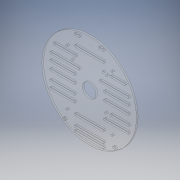
# Autodesk Inventor part: TopPlate
Saved by Autodesk Inventor 2018 (Build 220112000, 112)
## iProperties
Created: 2018-01-11
Part Number: TopPlate
Material: Polycarbonate, Clear
Document SubType Name: Modeling
Designer: Kyle
Density: 1.2 g/cm^3
Appearance: Polycarbonate - Clear
Author: Kyle
Autodesk Inventor part; units mm, degrees
ref_plane "YZ Plane" through (0, 0, 0) normal (1, 0, 0) x (0, 1, 0)
ref_plane "XZ Plane" through (0, 0, 0) normal (0, 1, 0) x (-1, 0, 0)
ref_plane "XY Plane" through (0, 0, 0) normal (0, 0, 1) x (1, 0, 0)
sketch "Sketch1" plane through (0, 0, 0) normal (0, 0, 1) x (1, 0, 0)
  circle A0 centre (0, 0) radius 69.85
  dimension "d0" = 139.7
  constraints: 1 centre point, 1 coincident
  measures "d0" diameter of A0
extrude "Extrusion1" add sketch "Sketch1" along normal blind 2.54
sketch "Sketch2" plane through (0, 0, 2.54) normal (0, 0, 1) x (1, 0, 0)
  circle A0 centre (0, 0) radius 10.16
  dimension "d3" = 20.32
  constraints: 1 centre point, 1 coincident
  measures "d3" diameter of A0
extrude "Extrusion2" cut sketch "Sketch2" against normal blind 2.54
sketch "Sketch3" plane through (0, 0, 2.54) normal (0, 0, 1) x (1, 0, 0)
  circle A0 centre (0, 0) radius 69.85 projected
  line L0 (-20.6375, 48.26) -> (20.6375, 48.26)
  line L1 (22.225, 46.6725) -> (22.225, 46.6725)
  line L2 (20.6375, 45.085) -> (-20.6375, 45.085)
  line L3 (-22.225, 46.6725) -> (-22.225, 46.6725)
  line L4 (14.9225, 63.5) -> (20.6375, 63.5)
  line L5 (22.225, 61.9125) -> (22.225, 61.9125)
  line L6 (20.6375, 60.325) -> (14.9225, 60.325)
  line L7 (13.335, 61.9125) -> (13.335, 61.9125)
  line L8 (-14.9225, 60.325) -> (-20.6375, 60.325)
  line L9 (-22.225, 61.9125) -> (-22.225, 61.9125)
  line L10 (-20.6375, 63.5) -> (-14.9225, 63.5)
  line L11 (-13.335, 61.9125) -> (-13.335, 61.9125)
  arc A1 (20.6375, 45.085) -> (22.225, 46.6725) centre (20.6375, 46.6725) ccw
  arc A2 (22.225, 46.6725) -> (20.6375, 48.26) centre (20.6375, 46.6725) ccw
  circle A3 centre (20.6375, 33.9725) radius 1.5875
  line L12 (32.7025, 35.56) -> (52.3875, 35.56)
  line L13 (53.975, 33.9725) -> (53.975, 33.9725)
  line L14 (52.3875, 32.385) -> (32.7025, 32.385)
  line L15 (31.115, 33.9725) -> (31.115, 33.9725)
  circle A4 centre (33.655, 40.9575) radius 1.5875
  circle A5 centre (25.7175, 32.0675) radius 1.5875
  circle A6 centre (-33.02, 40.9575) radius 1.5875
  line L16 (-51.7525, 35.56) -> (-20.6375, 35.56)
  line L17 (-19.05, 33.9725) -> (-19.05, 33.9725)
  line L18 (-20.6375, 32.385) -> (-51.7525, 32.385)
  line L19 (-53.34, 33.9725) -> (-53.34, 33.9725)
  arc A7 (-20.6375, 48.26) -> (-22.225, 46.6725) centre (-20.6375, 46.6725) ccw
  arc A8 (-22.225, 46.6725) -> (-20.6375, 45.085) centre (-20.6375, 46.6725) ccw
  arc A9 (-20.6375, 32.385) -> (-19.05, 33.9725) centre (-20.6375, 33.9725) ccw
  arc A10 (-19.05, 33.9725) -> (-20.6375, 35.56) centre (-20.6375, 33.9725) ccw
  circle A11 centre (-25.4, 26.3525) radius 1.5875
  arc A12 (-22.225, 61.9125) -> (-20.6375, 60.325) centre (-20.6375, 61.9125) ccw
  arc A13 (-20.6375, 63.5) -> (-22.225, 61.9125) centre (-20.6375, 61.9125) ccw
  arc A14 (-13.335, 61.9125) -> (-14.9225, 63.5) centre (-14.9225, 61.9125) ccw
  arc A15 (-14.9225, 60.325) -> (-13.335, 61.9125) centre (-14.9225, 61.9125) ccw
  arc A16 (14.9225, 63.5) -> (13.335, 61.9125) centre (14.9225, 61.9125) ccw
  arc A17 (13.335, 61.9125) -> (14.9225, 60.325) centre (14.9225, 61.9125) ccw
  arc A18 (20.6375, 60.325) -> (22.225, 61.9125) centre (20.6375, 61.9125) ccw
  arc A19 (22.225, 61.9125) -> (20.6375, 63.5) centre (20.6375, 61.9125) ccw
  arc A20 (-51.7525, 35.56) -> (-53.34, 33.9725) centre (-51.7525, 33.9725) ccw
  arc A21 (-53.34, 33.9725) -> (-51.7525, 32.385) centre (-51.7525, 33.9725) ccw
  arc A22 (32.7025, 35.56) -> (31.115, 33.9725) centre (32.7025, 33.9725) ccw
  arc A23 (31.115, 33.9725) -> (32.7025, 32.385) centre (32.7025, 33.9725) ccw
  arc A24 (52.3875, 32.385) -> (53.975, 33.9725) centre (52.3875, 33.9725) ccw
  arc A25 (53.975, 33.9725) -> (52.3875, 35.56) centre (52.3875, 33.9725) ccw
  line L20 (-56.8325, 21.59) -> (-15.5575, 21.59)
  line L21 (-13.97, 20.0025) -> (-13.97, 20.0025)
  line L22 (-15.5575, 18.415) -> (-56.8325, 18.415)
  line L23 (-58.42, 20.0025) -> (-58.42, 20.0025)
  line L24 (-57.15, 11.43) -> (-22.225, 11.43)
  line L25 (-20.6375, 9.8425) -> (-20.6375, 9.8425)
  line L26 (-22.225, 8.255) -> (-57.15, 8.255)
  line L27 (-58.7375, 9.8425) -> (-58.7375, 9.8425)
  line L28 (-57.15, 0) -> (-22.225, 0)
  line L29 (-20.6375, -1.5875) -> (-20.6375, -1.5875)
  line L30 (-22.225, -3.175) -> (-57.15, -3.175)
  line L31 (-58.7375, -1.5875) -> (-58.7375, -1.5875)
  line L32 (-57.15, -13.97) -> (-22.225, -13.97)
  line L33 (-20.6375, -15.5575) -> (-20.6375, -15.5575)
  line L34 (-22.225, -17.145) -> (-57.15, -17.145)
  line L35 (-58.7375, -15.5575) -> (-58.7375, -15.5575)
  line L36 (-57.15, -24.13) -> (-22.225, -24.13)
  line L37 (-20.6375, -25.7175) -> (-20.6375, -25.7175)
  line L38 (-22.225, -27.305) -> (-57.15, -27.305)
  line L39 (-58.7375, -25.7175) -> (-58.7375, -25.7175)
  arc A26 (-56.8325, 21.59) -> (-58.42, 20.0025) centre (-56.8325, 20.0025) ccw
  arc A27 (-58.42, 20.0025) -> (-56.8325, 18.415) centre (-56.8325, 20.0025) ccw
  arc A28 (-15.5575, 18.415) -> (-13.97, 20.0025) centre (-15.5575, 20.0025) ccw
  arc A29 (-13.97, 20.0025) -> (-15.5575, 21.59) centre (-15.5575, 20.0025) ccw
  arc A30 (-57.15, 11.43) -> (-58.7375, 9.8425) centre (-57.15, 9.8425) ccw
  arc A31 (-58.7375, 9.8425) -> (-57.15, 8.255) centre (-57.15, 9.8425) ccw
  arc A32 (-22.225, 8.255) -> (-20.6375, 9.8425) centre (-22.225, 9.8425) ccw
  arc A33 (-20.6375, 9.8425) -> (-22.225, 11.43) centre (-22.225, 9.8425) ccw
  arc A34 (-58.7375, -1.5875) -> (-57.15, -3.175) centre (-57.15, -1.5875) ccw
  arc A35 (-57.15, 0) -> (-58.7375, -1.5875) centre (-57.15, -1.5875) ccw
  arc A36 (-20.6375, -1.5875) -> (-22.225, 0) centre (-22.225, -1.5875) ccw
  arc A37 (-22.225, -3.175) -> (-20.6375, -1.5875) centre (-22.225, -1.5875) ccw
  arc A38 (-20.6375, -15.5575) -> (-22.225, -13.97) centre (-22.225, -15.5575) ccw
  arc A39 (-22.225, -17.145) -> (-20.6375, -15.5575) centre (-22.225, -15.5575) ccw
  arc A40 (-58.7375, -15.5575) -> (-57.15, -17.145) centre (-57.15, -15.5575) ccw
  arc A41 (-57.15, -13.97) -> (-58.7375, -15.5575) centre (-57.15, -15.5575) ccw
  arc A42 (-57.15, -24.13) -> (-58.7375, -25.7175) centre (-57.15, -25.7175) ccw
  arc A43 (-58.7375, -25.7175) -> (-57.15, -27.305) centre (-57.15, -25.7175) ccw
  arc A44 (-22.225, -27.305) -> (-20.6375, -25.7175) centre (-22.225, -25.7175) ccw
  arc A45 (-20.6375, -25.7175) -> (-22.225, -24.13) centre (-22.225, -25.7175) ccw
  arc A46 (22.733, -24.13) -> (21.1455, -25.7175) centre (22.733, -25.7175) ccw
  arc A47 (21.1455, -25.7175) -> (22.733, -27.305) centre (22.733, -25.7175) ccw
  line L40 (58.928, 20.0025) -> (58.928, 20.0025)
  arc A48 (21.1455, 9.8425) -> (22.733, 8.255) centre (22.733, 9.8425) ccw
  line L41 (22.733, -3.175) -> (57.658, -3.175)
  line L42 (57.658, 0) -> (22.733, 0)
  arc A49 (57.658, -3.175) -> (59.2455, -1.5875) centre (57.658, -1.5875) ccw
  arc A50 (59.2455, -1.5875) -> (57.658, 0) centre (57.658, -1.5875) ccw
  line L43 (22.733, 8.255) -> (57.658, 8.255)
  arc A51 (57.658, 8.255) -> (59.2455, 9.8425) centre (57.658, 9.8425) ccw
  line L44 (57.658, 11.43) -> (22.733, 11.43)
  arc A52 (59.2455, 9.8425) -> (57.658, 11.43) centre (57.658, 9.8425) ccw
  arc A53 (57.3405, 18.415) -> (58.928, 20.0025) centre (57.3405, 20.0025) ccw
  line L45 (16.0655, 18.415) -> (57.3405, 18.415)
  line L46 (57.3405, 21.59) -> (16.0655, 21.59)
  arc A54 (22.733, 11.43) -> (21.1455, 9.8425) centre (22.733, 9.8425) ccw
  arc A55 (21.1455, -1.5875) -> (22.733, -3.175) centre (22.733, -1.5875) ccw
  arc A56 (14.478, 20.0025) -> (16.0655, 18.415) centre (16.0655, 20.0025) ccw
  line L47 (21.1455, 9.8425) -> (21.1455, 9.8425)
  line L48 (14.478, 20.0025) -> (14.478, 20.0025)
  arc A57 (16.0655, 21.59) -> (14.478, 20.0025) centre (16.0655, 20.0025) ccw
  line L49 (21.1455, -25.7175) -> (21.1455, -25.7175)
  line L50 (59.2455, -25.7175) -> (59.2455, -25.7175)
  arc A58 (57.658, -27.305) -> (59.2455, -25.7175) centre (57.658, -25.7175) ccw
  line L51 (57.658, -24.13) -> (22.733, -24.13)
  line L52 (22.733, -27.305) -> (57.658, -27.305)
  line L53 (21.1455, -1.5875) -> (21.1455, -1.5875)
  arc A59 (22.733, 0) -> (21.1455, -1.5875) centre (22.733, -1.5875) ccw
  line L54 (59.2455, -15.5575) -> (59.2455, -15.5575)
  arc A60 (59.2455, -25.7175) -> (57.658, -24.13) centre (57.658, -25.7175) ccw
  line L55 (59.2455, -1.5875) -> (59.2455, -1.5875)
  line L56 (59.2455, 9.8425) -> (59.2455, 9.8425)
  arc A61 (58.928, 20.0025) -> (57.3405, 21.59) centre (57.3405, 20.0025) ccw
  line L57 (32.258, -17.145) -> (57.658, -17.145)
  line L58 (59.2455, -15.5575) -> (59.2455, -15.5575)
  line L59 (57.658, -13.97) -> (32.258, -13.97)
  line L60 (30.6705, -15.5575) -> (30.6705, -15.5575)
  arc A62 (30.6705, -15.5575) -> (32.258, -17.145) centre (32.258, -15.5575) ccw
  arc A63 (32.258, -13.97) -> (30.6705, -15.5575) centre (32.258, -15.5575) ccw
  arc A64 (57.658, -17.145) -> (59.2455, -15.5575) centre (57.658, -15.5575) ccw
  arc A65 (59.2455, -15.5575) -> (57.658, -13.97) centre (57.658, -15.5575) ccw
  circle A66 centre (24.3205, -16.8275) radius 1.5875
  circle A67 centre (33.655, -40.9575) radius 1.5875
  circle A68 centre (-33.02, -40.9575) radius 1.5875
  line L61 (-20.6375, -39.37) -> (20.6375, -39.37)
  line L62 (22.225, -40.9575) -> (22.225, -40.9575)
  line L63 (20.6375, -42.545) -> (-20.6375, -42.545)
  line L64 (-22.225, -40.9575) -> (-22.225, -40.9575)
  line L65 (-20.6375, -54.61) -> (20.6375, -54.61)
  line L66 (22.225, -56.1975) -> (22.225, -56.1975)
  line L67 (20.6375, -57.785) -> (-20.6375, -57.785)
  line L68 (-22.225, -56.1975) -> (-22.225, -56.1975)
  line L69 (-20.6375, -60.96) -> (20.6375, -60.96)
  line L70 (22.225, -62.5475) -> (22.225, -62.5475)
  line L71 (20.6375, -64.135) -> (-20.6375, -64.135)
  line L72 (-22.225, -62.5475) -> (-22.225, -62.5475)
  line L73 (35.8775, -53.34) -> (37.7825, -53.34)
  line L74 (39.37, -54.9275) -> (39.37, -54.9275)
  line L75 (37.7825, -56.515) -> (35.8775, -56.515)
  line L76 (34.29, -54.9275) -> (34.29, -54.9275)
  line L77 (-37.7825, -53.34) -> (-35.8775, -53.34)
  line L78 (-34.29, -54.9275) -> (-34.29, -54.9275)
  line L79 (-35.8775, -56.515) -> (-37.7825, -56.515)
  line L80 (-39.37, -54.9275) -> (-39.37, -54.9275)
  arc A69 (-20.6375, -39.37) -> (-22.225, -40.9575) centre (-20.6375, -40.9575) ccw
  arc A70 (-22.225, -40.9575) -> (-20.6375, -42.545) centre (-20.6375, -40.9575) ccw
  arc A71 (20.6375, -42.545) -> (22.225, -40.9575) centre (20.6375, -40.9575) ccw
  arc A72 (22.225, -40.9575) -> (20.6375, -39.37) centre (20.6375, -40.9575) ccw
  arc A73 (22.225, -56.1975) -> (20.6375, -54.61) centre (20.6375, -56.1975) ccw
  arc A74 (20.6375, -57.785) -> (22.225, -56.1975) centre (20.6375, -56.1975) ccw
  arc A75 (-22.225, -56.1975) -> (-20.6375, -57.785) centre (-20.6375, -56.1975) ccw
  arc A76 (-20.6375, -54.61) -> (-22.225, -56.1975) centre (-20.6375, -56.1975) ccw
  arc A77 (-22.225, -62.5475) -> (-20.6375, -64.135) centre (-20.6375, -62.5475) ccw
  arc A78 (-20.6375, -60.96) -> (-22.225, -62.5475) centre (-20.6375, -62.5475) ccw
  arc A79 (22.225, -62.5475) -> (20.6375, -60.96) centre (20.6375, -62.5475) ccw
  arc A80 (20.6375, -64.135) -> (22.225, -62.5475) centre (20.6375, -62.5475) ccw
  arc A81 (34.29, -54.9275) -> (35.8775, -56.515) centre (35.8775, -54.9275) ccw
  arc A82 (35.8775, -53.34) -> (34.29, -54.9275) centre (35.8775, -54.9275) ccw
  arc A83 (39.37, -54.9275) -> (37.7825, -53.34) centre (37.7825, -54.9275) ccw
  arc A84 (37.7825, -56.515) -> (39.37, -54.9275) centre (37.7825, -54.9275) ccw
  arc A85 (-35.8775, -56.515) -> (-34.29, -54.9275) centre (-35.8775, -54.9275) ccw
  arc A86 (-34.29, -54.9275) -> (-35.8775, -53.34) centre (-35.8775, -54.9275) ccw
  arc A87 (-37.7825, -53.34) -> (-39.37, -54.9275) centre (-37.7825, -54.9275) ccw
  arc A88 (-39.37, -54.9275) -> (-37.7825, -56.515) centre (-37.7825, -54.9275) ccw
  point P0 (0, 69.85)
  point P1 (69.85, 0)
  point P2 (0, -69.85)
  point P3 (-69.85, 0)
  point P4 (22.225, 45.085)
  point P5 (22.225, 48.26)
  point P6 (-22.225, 45.085)
  point P7 (22.225, 60.325)
  point P8 (22.225, 63.5)
  point P9 (13.335, 60.325)
  point P10 (-13.335, 60.325)
  point P11 (-22.225, 63.5)
  point P12 (-22.225, 60.325)
  point P13 (53.975, 32.385)
  point P14 (53.975, 35.56)
  point P15 (31.115, 32.385)
  point P16 (-19.05, 32.385)
  point P17 (-19.05, 35.56)
  point P18 (-53.34, 32.385)
  point P19 (-13.97, 18.415)
  point P20 (-13.97, 21.59)
  point P21 (-58.42, 18.415)
  point P22 (-20.6375, 8.255)
  point P23 (-20.6375, 11.43)
  point P24 (-58.7375, 8.255)
  point P25 (-20.6375, -3.175)
  point P26 (-20.6375, 0)
  point P27 (-58.7375, -3.175)
  point P28 (-20.6375, -17.145)
  point P29 (-20.6375, -13.97)
  point P30 (-58.7375, -17.145)
  point P31 (-20.6375, -27.305)
  point P32 (-20.6375, -24.13)
  point P33 (-58.7375, -27.305)
  point P34 (14.478, 20.0025)
  point P35 (59.2455, -3.175)
  point P36 (59.2455, 8.255)
  point P37 (58.928, 18.415)
  point P38 (21.1455, -24.13)
  point P39 (30.6705, -17.145)
  point P40 (21.1455, 0)
  point P41 (21.1455, 8.255)
  point P42 (14.478, 18.415)
  point P43 (14.478, 21.59)
  point P44 (21.1455, -27.305)
  point P45 (59.2455, -27.305)
  point P46 (21.1455, -3.175)
  point P47 (59.2455, -17.145)
  point P48 (21.1455, 11.43)
  point P49 (30.6705, -17.145)
  point P50 (-22.225, -39.37)
  point P51 (22.225, -39.37)
  point P52 (-22.225, -54.61)
  point P53 (22.225, -54.61)
  point P54 (-22.225, -60.96)
  point P55 (22.225, -60.96)
  point P56 (34.29, -53.34)
  point P57 (39.37, -56.515)
  point P58 (39.37, -53.34)
  point P59 (-39.37, -53.34)
  point P60 (-34.29, -53.34)
  dimension "d6" = 44.45
  dimension "d7" = 3.175
  dimension "d8" = 22.225
  dimension "d9" = 21.59
  dimension "d10" = 8.89
  dimension "d11" = 8.89
  dimension "d12" = 3.175
  dimension "d13" = 3.175
  dimension "d14" = 12.065
  dimension "d15" = 12.065
  dimension "d16" = 1.5875
  dimension "d17" = 3.175
  dimension "d18" = 11.1125
  dimension "d19" = 3.175
  dimension "d20" = 22.86
  dimension "d21" = 10.4775
  dimension "d22" = 3.175
  dimension "d23" = 5.3975
  dimension "d24" = 2.54
  dimension "d25" = 3.175
  dimension "d26" = 5.08
  dimension "d27" = 1.905
  dimension "d28" = 3.175
  dimension "d29" = 3.175
  dimension "d30" = 34.29
  dimension "d31" = 1.5875
  dimension "d32" = 1.5875
  dimension "d33" = 1.5875
  dimension "d34" = 0
  dimension "d35" = 13.97
  dimension "d36" = 3.175
  dimension "d37" = 6.0325
  dimension "d38" = 6.35
  dimension "d39" = 1.5875
  dimension "d40" = 3.175
  dimension "d41" = 44.45
  dimension "d42" = 5.08
  dimension "d43" = 10.795
  dimension "d44" = 3.175
  dimension "d45" = 38.1
  dimension "d46" = 6.985
  dimension "d47" = 3.175
  dimension "d48" = 38.1
  dimension "d49" = 3.175
  dimension "d50" = 38.1
  dimension "d51" = 3.175
  dimension "d52" = 38.1
  dimension "d53" = 8.255
  dimension "d54" = 10.795
  dimension "d55" = 6.985
  dimension "d56" = 1.5875
  dimension "d57" = 28.448
  dimension "d74" = 28.575
  dimension "d75" = 1.5875
  dimension "d76" = 3.175
  dimension "d77" = 6.35
  dimension "d78" = 1.27
  dimension "d79" = 44.45
  dimension "d80" = 22.225
  dimension "d81" = 44.45
  dimension "d82" = 44.45
  dimension "d83" = 39.37
  dimension "d84" = 12.065
  dimension "d85" = 3.175
  constraints: 164 point on circle, 162 end point, 128 tangent, 109 point on line, 88 centre point, 56 equal radius, 32 parallel, 16 horizontal, 16 perpendicular, 2 collinear, 2 symmetric about line, 1 coincident, 1 vertical, 7 other
  measures "d6" distance of point (22.225, 45.085) point (-22.225, 45.085)
  measures "d7" distance of point (22.225, 48.26) point (22.225, 45.085)
  measures "d8" distance from line of A0.start L1
  measures "d9" distance from line of A0.start L0
  measures "d10" distance of point (22.225, 60.325) point (13.335, 60.325)
  measures "d11" distance of point (-13.335, 60.325) point (-22.225, 60.325)
  measures "d12" distance of point (-22.225, 60.325) point (-22.225, 63.5)
  measures "d13" distance of point (22.225, 63.5) point (22.225, 60.325)
  measures "d14" distance between parallel lines of L0 L6
  measures "d15" distance between parallel lines of L8 L0
  measures "d16" radius of A1
  measures "d17" diameter of A3
  measures "d18" distance from line of A3.centre L2
  measures "d19" distance of point (53.975, 35.56) point (53.975, 32.385)
  measures "d20" distance of point (53.975, 32.385) point (31.115, 32.385)
  measures "d21" distance from line of A3.centre L15
  measures "d22" diameter of A4
  measures "d23" distance from line of A4.centre L12
  measures "d24" distance from line of L15 A4.centre
  measures "d25" diameter of A5
  measures "d26" horizontal distance of A3.centre A5.centre
  measures "d27" vertical distance of A3.centre A5.centre
  measures "d28" diameter of A6
  measures "d29" distance of point (-19.05, 35.56) point (-19.05, 32.385)
  measures "d30" distance of point (-19.05, 32.385) point (-53.34, 32.385)
  measures "d31" radius of A7
  measures "d32" radius of A9
  measures "d33" radius of A10
  measures "d34" horizontal distance of A10.centre A8.centre
  measures "d35" horizontal distance of A6.centre L17.start
  measures "d36" diameter of A11
  measures "d37" distance from line of L18 A11.centre
  measures "d38" horizontal distance of A11.centre L17.start
  measures "d39" radius of A12
  measures "d40" distance of point (-13.97, 21.59) point (-13.97, 18.415)
  measures "d41" distance of point (-13.97, 18.415) point (-58.42, 18.415)
  measures "d42" distance from line of L19.start L23
  measures "d43" distance between parallel lines of L18 L20
  measures "d44" distance of point (-20.637, 11.43) point (-20.637, 8.255)
  measures "d45" distance of point (-20.637, 8.255) point (-58.737, 8.255)
  measures "d46" distance between parallel lines of L22 L24
  measures "d47" distance of point (-20.637, 0) point (-20.637, -3.175)
  measures "d48" distance of point (-20.637, -3.175) point (-58.737, -3.175)
  measures "d49" distance of point (-20.637, -13.97) point (-20.637, -17.145)
  measures "d50" distance of point (-20.637, -17.145) point (-58.737, -17.145)
  measures "d51" distance of point (-20.637, -24.13) point (-20.637, -27.305)
  measures "d52" distance of point (-20.637, -27.305) point (-58.737, -27.305)
  measures "d53" distance between parallel lines of L28 L26
  measures "d54" distance between parallel lines of L30 L32
  measures "d55" distance between parallel lines of L36 L34
  measures "d56" radius of A26
  measures "d57" distance of L21.end point (14.478, 20.003)
  measures "d74" distance between parallel lines of L60 L58
  measures "d75" radius of A62
  measures "d76" diameter of A66
  measures "d77" horizontal distance of L60.end A66.centre
  measures "d78" vertical distance of A66.centre A62.centre
  measures "d79" distance of point (-22.225, -39.37) point (22.225, -39.37)
  measures "d80" distance from line of L62 point (0, 0)
  measures "d81" distance of point (-22.225, -54.61) point (22.225, -54.61)
  measures "d82" distance of point (-22.225, -60.96) point (22.225, -60.96)
  measures "d83" distance from line of L61 point (0, 0)
  measures "d84" distance between parallel lines of L65 L63
  measures "d85" distance between parallel lines of L69 L67
extrude "Extrusion3" cut sketch "Sketch3" against normal blind 2.54 contours L0 A2 A1 L2 A8 A7 | L4 A19 A18 L6 A17 A16 | L8 A12 A13 L10 A14 A15 | A3 | L12 A25 A24 L14 A23 A22 | A4 | A5 | A6 | L16 A10 A9 L18 A21 A20 | A11 | L20 A29 A28 L22 A27 A26 | L24 A33 A32 L26 A31 A30 | L28 A36 A37 L30 A34 A35 | L32 A38 A39 L34 A40 A41 | L36 A45 A44 L38 A43 A42 | L51 A60 A58 L52 A47 A46 | A54 L44 A52 A51 L43 A48 | A55 A59 L42 A50 A49 L41 | L45 A56 A57 L46 A61 A53 | A62 A63 L59 A65 A64 L57 | A66 | A67 | A68 | L61 A72 A71 L63 A70 A69 | L65 A73 A74 L67 A75 A76 | L69 A79 A80 L71 A77 A78 | L73 A83 A84 L75 A81 A82 | L77 A86 A85 L79 A88 A87
body "Solid1"
